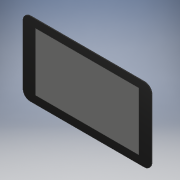
# Autodesk Inventor part: Touchscreen
Saved by Autodesk Inventor 2018 (Build 220112000, 112)
## iProperties
Created: 2018-03-22
Part Number: Touchscreen
Material: Generic
Document SubType Name: Modeling
Designer: brutu
Density: 1 g/cm^3
Appearance: Light Gray
Author: brutu
Autodesk Inventor part; units mm, degrees
ref_plane "YZ Plane" through (0, 0, 0) normal (1, 0, 0) x (0, 1, 0)
ref_plane "XZ Plane" through (0, 0, 0) normal (0, 1, 0) x (-1, 0, 0)
ref_plane "XY Plane" through (0, 0, 0) normal (0, 0, 1) x (1, 0, 0)
sketch "Sketch1" plane through (0, 0, 0) normal (0, 0, 1) x (1, 0, 0)
  line L0 (-85.48, 55.38) -> (85.48, 55.38)
  line L1 (96.48, 44.38) -> (96.48, -44.38)
  line L2 (85.48, -55.38) -> (-85.48, -55.38)
  line L3 (-96.48, -44.38) -> (-96.48, 44.38)
  arc A0 (-85.48, 55.38) -> (-96.48, 44.38) centre (-85.48, 44.38) ccw
  arc A1 (96.48, 44.38) -> (85.48, 55.38) centre (85.48, 44.38) ccw
  arc A2 (85.48, -55.38) -> (96.48, -44.38) centre (85.48, -44.38) ccw
  arc A3 (-96.48, -44.38) -> (-85.48, -55.38) centre (-85.48, -44.38) ccw
  point P0 (0, 0)
  point P1 (-96.48, 55.38)
  point P2 (96.48, 55.38)
  point P3 (-96.48, -55.38)
  dimension "d0" = 192.96
  dimension "d1" = 110.76
  dimension "d2" = 96.48
  dimension "d3" = 55.38
  dimension "d6" = 11
  constraints: 8 end point, 8 point on circle, 8 tangent, 6 point on line, 4 centre point, 3 equal radius, 2 parallel, 1 horizontal, 1 perpendicular
  measures "d0" distance of point (-96.48, 55.38) point (96.48, 55.38)
  measures "d1" distance of point (-96.48, -55.38) point (-96.48, 55.38)
  measures "d2" distance from line of point (0, 0) L3
  measures "d3" distance from line of L0 point (0, 0)
  measures "d6" radius of A0
extrude "Extrusion2" add sketch "Sketch1" along normal blind 1
sketch "Sketch3" plane through (0, 0, 0) normal (0, 0, -1) x (-1, 0, 0)
  line L0 (-83.1, 48.75) -> (83.1, 48.75)
  line L1 (83.1, 48.75) -> (83.1, -51.85)
  line L2 (83.1, -51.85) -> (-83.1, -51.85)
  line L3 (-83.1, -51.85) -> (-83.1, 48.75)
  line L4 (85.48, 55.38) -> (-85.48, 55.38) projected
  point P0 (0, 0)
  dimension "d9" = 166.2
  dimension "d10" = 100.6
  dimension "d12" = 83.1
  dimension "d13" = 6.63
  constraints: 8 end point, 2 parallel, 1 horizontal, 1 perpendicular
  measures "d9" distance of L0.start L0.end
  measures "d10" distance of L0.end L1.end
  measures "d12" distance from line of L1 point (0, 0)
  measures "d13" distance between parallel lines of L4 L0
extrude "Extrusion3" add sketch "Sketch3" along normal blind 4.96
sketch "Sketch4" plane through (0, 0, -4.96) normal (0, 0, -1) x (-1, 0, 0)
  line L0 (-70.6, 37.8) -> (-55.6, 37.8)
  line L1 (-55.6, 37.8) -> (-55.6, 29.8)
  line L2 (-55.6, 29.8) -> (-70.6, 29.8)
  line L3 (-70.6, 29.8) -> (-70.6, 37.8)
  circle A0 centre (-63.1, 33.8) radius 1.5
  line L4 (-83.1, 48.75) -> (-83.1, -51.85) projected
  line L5 (55.6, 37.8) -> (70.6, 37.8)
  circle A1 centre (63.1, 33.8) radius 1.5
  line L6 (55.6, 29.8) -> (55.6, 37.8)
  line L7 (70.6, 29.8) -> (55.6, 29.8)
  line L8 (70.6, 37.8) -> (70.6, 29.8)
  line L9 (-70.6, -27.85) -> (-55.6, -27.85)
  circle A2 centre (-63.1, -31.85) radius 1.5
  line L10 (-70.6, -35.85) -> (-70.6, -27.85)
  line L11 (-55.6, -35.85) -> (-70.6, -35.85)
  line L12 (-55.6, -27.85) -> (-55.6, -35.85)
  line L13 (55.6, -27.85) -> (70.6, -27.85)
  circle A3 centre (63.1, -31.85) radius 1.5
  line L14 (55.6, -35.85) -> (55.6, -27.85)
  line L15 (70.6, -35.85) -> (55.6, -35.85)
  line L16 (70.6, -27.85) -> (70.6, -35.85)
  line L17 (83.1, 48.75) -> (-83.1, 48.75) projected
  line L18 (-38.65, 20.45) -> (-38.65, 35.45)
  circle A4 centre (-34.65, 27.95) radius 1.25
  line L19 (-30.65, 20.45) -> (-38.65, 20.45)
  line L20 (-30.65, 35.45) -> (-30.65, 20.45)
  line L21 (-38.65, 35.45) -> (-30.65, 35.45)
  line L22 (83.1, -51.85) -> (83.1, 48.75) projected
  line L23 (85.48, 55.38) -> (-85.48, 55.38) projected
  line L24 (19.35, 20.45) -> (19.35, 35.45)
  line L25 (19.35, 35.45) -> (27.35, 35.45)
  line L26 (27.35, 35.45) -> (27.35, 20.45)
  line L27 (27.35, 20.45) -> (19.35, 20.45)
  circle A5 centre (23.35, 27.95) radius 1.25
  line L28 (-38.65, -28.55) -> (-38.65, -13.55)
  line L29 (-38.65, -13.55) -> (-30.65, -13.55)
  line L30 (-30.65, -13.55) -> (-30.65, -28.55)
  line L31 (-30.65, -28.55) -> (-38.65, -28.55)
  circle A6 centre (-34.65, -21.05) radius 1.25
  line L32 (19.35, -28.55) -> (19.35, -13.55)
  line L33 (19.35, -13.55) -> (27.35, -13.55)
  line L34 (27.35, -13.55) -> (27.35, -28.55)
  line L35 (27.35, -28.55) -> (19.35, -28.55)
  circle A7 centre (23.35, -21.05) radius 1.25
  point P0 (0, 0)
  point P1 (-55.6, 33.8)
  point P2 (-63.1, 37.8)
  point P3 (63.1, 37.8)
  point P4 (70.6, 33.8)
  point P5 (-63.1, -27.85)
  point P6 (-55.6, -31.85)
  point P7 (63.1, -27.85)
  point P8 (70.6, -31.85)
  point P9 (64.6875, 33.5375)
  point P10 (72.1875, 29.5375)
  point P11 (-38.65, 27.95)
  point P12 (-34.65, 35.45)
  point P13 (122.6875, 33.5375)
  point P14 (19.35, 27.95)
  point P15 (130.1875, 29.5375)
  point P16 (23.35, 35.45)
  point P17 (64.6875, -15.4625)
  point P18 (-38.65, -21.05)
  point P19 (72.1875, -19.4625)
  point P20 (-34.65, -13.55)
  point P21 (122.6875, -15.4625)
  point P22 (19.35, -21.05)
  point P23 (130.1875, -19.4625)
  point P24 (23.35, -13.55)
  dimension "d16" = 15
  dimension "d17" = 8
  dimension "d18" = 3
  dimension "d19" = 20
  dimension "d22" = 126.2
  dimension "d25" = 65.65
  dimension "d29" = 2.5
  dimension "d30" = 20.8
  dimension "d32" = 48.45
  dimension "d33" = 21.58
  dimension "d44" = 58
  dimension "d47" = 49
  constraints: 48 end point, 9 vertical, 8 centre point, 6 horizontal, 3 perpendicular, 2 horizontal alignment, 2 midpoint, 2 parallel, 2 vertical alignment, 1 collinear, 97 other
  measures "d16" distance of L0.start L0.end
  measures "d17" distance of L0.end L1.end
  measures "d18" diameter of A0
  measures "d19" distance from line of L4 A0.centre
  measures "d22" distance of L0.start L5.start
  measures "d25" distance of L0.start L9.start
  measures "d29" diameter of A4
  measures "d30" distance from line of L17 A4.centre
  measures "d32" distance from line of L4 A4.centre
  measures "d33" distance from line of L23 A0.centre
  measures "d44" distance of L19.end L27.end
  measures "d47" distance of L19.end L31.end
extrude "Extrusion4" add sketch "Sketch4" along normal blind 2.5
chamfer "Chamfer1" distance 2.5 angle 45 16 edges at (70.6, 33.8, -7.46) (55.6, 33.8, -7.46) (34.65, 35.45, -7.46) (34.65, 20.45, -7.46) (-23.35, 35.45, -7.46) (-23.35, 20.45, -7.46) (-55.6, 33.8, -7.46) (-70.6, 33.8, -7.46) (70.6, -31.85, -7.46) (55.6, -31.85, -7.46) (34.65, -13.55, -7.46) (34.65, -28.55, -7.46) (-23.35, -13.55, -7.46) (-23.35, -28.55, -7.46) (-55.6, -31.85, -7.46) (-70.6, -31.85, -7.46)
sketch "Sketch5" plane through (0, 0, 1) normal (0, 0, 1) x (1, 0, 0)
  line L0 (-77.5, 43.5) -> (77.5, 43.5)
  line L1 (77.5, 43.5) -> (77.5, -43.5)
  line L2 (77.5, -43.5) -> (-77.5, -43.5)
  line L3 (-77.5, -43.5) -> (-77.5, 43.5)
  point P0 (0, 0)
  dimension "d55" = 155
  dimension "d56" = 87
  dimension "d57" = 43.5
  dimension "d58" = 77.5
  constraints: 8 end point, 2 parallel, 1 horizontal, 1 perpendicular
  measures "d55" distance of L0.start L0.end
  measures "d56" distance of L2.end L0.start
  measures "d57" distance from line of point (0, 0) L0
  measures "d58" distance from line of L3 point (0, 0)
extrude "Extrusion5" add sketch "Sketch5" along normal blind 0.01
equation "\"d2\" = 0.5 * d0"
equation "\"d3\" = 0.5 * d1"
equation "\"d12\" = 0.5 * d9"
equation "\"d57\" = 0.5 * d56"
equation "\"d58\" = 0.5 * d55"
body "Solid2"
